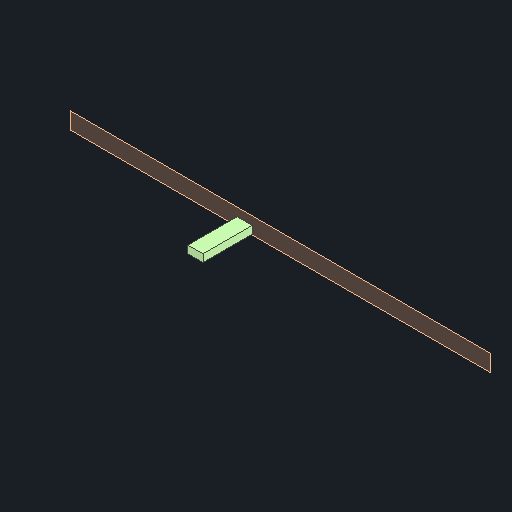
# Autodesk Inventor part: 2x4x13
Saved by Autodesk Inventor 2027 (Build 310192000, 192)
## iProperties
Created: 2026-08-07
Part Number: 2x4x13
Material: Generic
Document SubType Name: Modeling
Designer: lucas
Density: 1 g/cm^3
Appearance: Default
Author: lucas
Autodesk Inventor part; units mm, degrees
ref_plane "YZ Plane" through (0, 0, 0) normal (1, 0, 0) x (0, 1, 0)
ref_plane "XZ Plane" through (0, 0, 0) normal (0, 1, 0) x (-1, 0, 0)
ref_plane "XY Plane" through (0, 0, 0) normal (0, 0, 1) x (1, 0, 0)
ref_plane "Work Plane1" through (0, 0, 0) normal (0, 0, 1) x (1, 0, 0)
sketch "Sketch1" plane through (0, 0, 0) normal (0, 0, 1) x (1, 0, 0)
  line L0 (-190.5, 0) -> (-190.5, -50.8) projected
  line L1 (-291.8938, 0) -> (-190.5, 0) projected
  line L2 (-291.8938, -50.8) -> (-190.5, -50.8)
  line L3 (-291.8938, 0) -> (-291.8938, -50.8) projected
  line L4 (-190.5, 0) -> (-291.8938, 0)
  line L5 (-291.8938, 0) -> (-291.8938, -50.8)
  line L6 (-291.8938, -50.8) -> (-190.5, -50.8)
  line L7 (-190.5, -50.8) -> (-190.5, 0)
  point P0 (0, 0)
  constraints: 10 end point, 2 horizontal, 2 parallel, 1 perpendicular, 1 other
extrude "Extrusion1" add sketch "Sketch1" along normal blind 330.2
body "Solid1"
